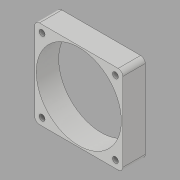
# Autodesk Inventor part: Fan
Saved by Autodesk Inventor 2017 (Build 210142000, 142)
## iProperties
Created: 2022-09-19
Part Number: Fan
Material: Generic
Document SubType Name: Modeling
Designer: JTS
Density: 1 g/cm^3
Appearance: Default
Author: JTS
Autodesk Inventor part; units mm, degrees
ref_plane "YZ Plane" through (0, 0, 0) normal (1, 0, 0) x (0, 1, 0)
ref_plane "XZ Plane" through (0, 0, 0) normal (0, 1, 0) x (-1, 0, 0)
ref_plane "XY Plane" through (0, 0, 0) normal (0, 0, 1) x (1, 0, 0)
sketch "Sketch1" plane through (0, 0, 0) normal (0, 0, 1) x (1, 0, 0)
  line L0 (-30, -30) -> (30, -30)
  line L1 (30, -30) -> (30, 30)
  line L2 (30, 30) -> (-30, 30)
  line L3 (-30, 30) -> (-30, -30)
  line L4 (-30, -30) -> (30, 30) construction
  line L5 (30, -30) -> (-30, 30) construction
  circle A0 centre (0, 0) radius 29
  circle A1 centre (-25, 25) radius 2
  circle A2 centre (25, 25) radius 2
  circle A3 centre (25, -25) radius 2
  circle A4 centre (-25, -25) radius 2
  line L6 (-25, 25) -> (25, 25) construction
  line L7 (25, 25) -> (25, -25) construction
  line L8 (25, -25) -> (-25, -25) construction
  dimension "d0" = 60
  dimension "d3" = 50
  dimension "d4" = 4
  dimension "d5" = 58
  constraints: 18 end point, 5 centre point, 4 horizontal, 4 point on line, 3 equal radius, 3 vertical, 2 midpoint, 1 coincident, 1 perpendicular
  measures "d0" distance of L2.end L0.start
  measures "d3" distance of L6.end L7.end
  measures "d4" diameter of A1
  measures "d5" diameter of A0
extrude "Extrusion1" add sketch "Sketch1" along normal blind 15.3
fillet "Fillet1" radius 3.175 4 edges at (30, 30, 7.65) (30, -30, 7.65) (-30, 30, 7.65) (-30, -30, 7.65)
body "Solid1"
